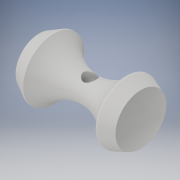
# Autodesk Inventor part: A
Saved by Autodesk Inventor 2017 (Build 210142000, 142)
## iProperties
Part Number: A
Material: 一般
Document SubType Name: Modeling
Designer: user
Density: 1 g/cm^3
Appearance: 預設
Author: user
Autodesk Inventor part; units mm, degrees
ref_plane "YZ Plane" through (0, 0, 0) normal (1, 0, 0) x (0, 1, 0)
ref_plane "XZ Plane" through (0, 0, 0) normal (0, 1, 0) x (-1, 0, 0)
ref_plane "XY Plane" through (0, 0, 0) normal (0, 0, 1) x (1, 0, 0)
sketch "草圖1" plane through (0, 0, 0) normal (0, 0, 1) x (1, 0, 0)
  line L0 (0, 18.5) -> (10, 24)
  line L1 (10, 24) -> (11.5, 24)
  line L2 (80, 20) -> (70, 24)
  line L3 (70, 24) -> (68.5, 24)
  line L4 (0, 0) -> (80, 0)
  arc A0 (11.5, 24) -> (68.5, 24) centre (40, 44.3162) ccw
  arc A1 (4.5352, 0) -> (0, 18.5) centre (-35.4648, 0) ccw
  arc A2 (80, 20) -> (75.8258, 0) centre (125.8258, 0) ccw
  dimension "d0" = 18.5
  dimension "d2" = 1.5
  dimension "d3" = 1.5
  dimension "d4" = 24
  dimension "d6" = 20
  dimension "d8" = 24
  dimension "d9" = 35
  dimension "d21" = 40
  dimension "d23" = 50
  dimension "d33" = 158.199
  dimension "d34" = 129.388
  dimension "d35" = 48.2808
  dimension "d36" = 16.21
  dimension "d37" = 1.5503
  dimension "d38" = 24
  dimension "d39" = 46.5964
  constraints: 10 end point, 6 point on circle, 3 centre point, 2 point on line, 1 horizontal, 1 parallel
  measures "d0" distance of L4.start L0.start
  measures "d2" distance of L0.end L1.end
  measures "d3" distance of L2.end L3.end
  measures "d4" distance between parallel lines of L1 L4
  measures "d6" distance of L4.end L2.start
  measures "d8" distance from line of L3.end L4
  measures "d9" radius of A0
  measures "d21" radius of A1
  measures "d23" radius of A2
  measures "d33" angle of L2 L3
  measures "d34" angle of L2 L0
  measures "d35" distance from line of L4.start L2
  measures "d36" distance from line of L4.start L0
  measures "d37" distance from line of A2.centre L2
  measures "d38" distance from line of A2.centre L3
  measures "d39" distance from line of A1.start L2
revolve "迴轉1" add sketch "草圖1" angle 360 about axis through (0, 0, 0) along (1, 0, 0)
sketch "草圖2" plane through (0, 0, 0) normal (0, 1, 0) x (-1, 0, 0)
  circle A0 centre (-40, 0) radius 5
  point P0 (0, 0)
  dimension "d11" = 10
  dimension "d12" = 0
  dimension "d13" = 40
  constraints: 1 centre point
  measures "d11" diameter of A0
  measures "d12" vertical distance of A0.centre point (0, 0)
  measures "d13" distance of point (0, 0) A0.centre
extrude "擠出1" cut sketch "草圖2" along normal mid plane 60
